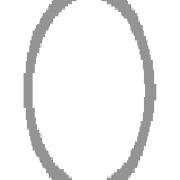
# Autodesk Inventor part: 4130_1x0.065
Saved by Autodesk Inventor 2021 (Build 250183000, 183)
## iProperties
Created: 2020-11-09
Part Number: 4130_1x0.065
Material: Steel, Alloy
Document SubType Name: Modeling
Designer: qv17m
Language: en-US
Size Designation: (Unnamed 1)
Categories: <MemberInstance><Categories><Category DisplayName="Structural Shapes" InternalName="089c4875-fa83-4c05-b084-43b9cc11f5ed" Mnemonic="GRDR"><CategoryParameter DisplayName="Mass per Length Unit" InternalName="0bb95a10-148f-4027-a459-38d7b056702a" Mnemonic="shpmass"/><CategoryParameter DisplayName="Section Area" InternalName="1ff91680-64b0-4202-b9a3-7fd3f94bba3b" Mnemonic="secarea"/><CategoryParameter DisplayName="Radius of Gyration (x)" InternalName="25778675-03e9-40c1-b6a8-4a9ed693320d" Mnemonic="gyrradx"/><CategoryParameter DisplayName="Torsional Rigidity Modulus" InternalName="26c1ec35-5026-4c63-ad0a-751cf684a536" Mnemonic="torrigmod"/><CategoryParameter DisplayName="Distance of the Center of Gravity X-X" InternalName="26c9bdb8-9c79-4b4f-a92e-8e197583c9c4" Mnemonic="grcendistX"/><CategoryParameter DisplayName="Legacy Member ID" InternalName="340afe4f-75d7-48d3-ab7d-943f3c3da468" Mnemonic="LegacyMemberID"/><CategoryParameter DisplayName="Base Length" InternalName="42e34263-8f20-4d0e-ad48-bf1385b87c24" Mnemonic="shplen"/><CategoryParameter DisplayName="Moment of Inertia (y)" InternalName="4b9f58ea-bced-460e-81ea-3d29ca5a49e3" Mnemonic="inermomy"/><CategoryParameter DisplayName="Moment of Inertia (x)" InternalName="4cd780bc-73d7-43ac-917a-579e5cbd684d" Mnemonic="inermomx"/><CategoryParameter DisplayName="Custom Base Point" InternalName="4f1d1b73-316d-484b-a3df-9cbabb16eb77" Mnemonic="shpBasePoint"/><CategoryParameter DisplayName="Shape Height" InternalName="50274e7d-5ac0-4796-92cb-c59e54983c67" Mnemonic="shpheig"/><CategoryParameter DisplayName="Section Module (y)" InternalName="59eaa5e9-d227-48dc-b6c1-6920f96e0f95" Mnemonic="secmody"/><CategoryParameter DisplayName="Section Designation" InternalName="5a64d034-428d-49c8-ba32-7619764de20f" Mnemonic="shpdes"/><CategoryParameter DisplayName="Section Module (x)" InternalName="72cfad18-cf51-4ed4-aaa7-c6b224f8419f" Mnemonic="secmodx"/><CategoryParameter DisplayName="Torsional Section Modulus" InternalName="7c55a8dc-8844-49f9-a867-cc677b30ec9a" Mnemonic="torsecmod"/><CategoryParameter DisplayName="Shape Width" InternalName="7c717d54-a18f-4666-b4d4-573cce22c62c" Mnemonic="shpwdth"/><CategoryParameter DisplayName="Second Shape Thickness" InternalName="9251a8e1-85fd-4e47-af99-afdb762317d9" Mnemonic="shpthick2"/><CategoryParameter DisplayName="FG Authored" InternalName="9c666724-f362-4ea7-ac62-f6a007de5c69" Mnemonic="shpFGAuto"/><CategoryParameter DisplayName="Distance of the Center of Gravity Y-Y" InternalName="bcc4fb17-7af4-436a-8f8c-d0aa3b0248c5" Mnemonic="grcendistY"/><CategoryParameter DisplayName="Radius of Gyration (y)" InternalName="bfa18ebe-1636-4dbe-8d42-b263e0b73184" Mnemonic="gyrrady"/><CategoryParameter DisplayName="Shape Thickness" InternalName="d109cf76-8eb4-42fc-9800-4409734adc67" Mnemonic="shpthick"/><CategoryParameter DisplayName="Coefficient of Shear Displacement" InternalName="de4c90c6-aaa8-468f-a335-6737b311b5d3" Mnemonic="shdispc"/><Category DisplayName="Round Tubes" InternalName="992db413-5889-4444-87eb-da7d0d4daf07" Mnemonic="TBSHP"><CategoryParameter DisplayName="Radius of Gyration (x)" InternalName="3dee80f9-25b5-4b66-b49a-b691523a1a28" Mnemonic="gyrradx"/><CategoryParameter DisplayName="Section Module (x)" InternalName="60bb9a9e-a6fd-4017-9231-e997b611324d" Mnemonic="secmodx"/><CategoryParameter DisplayName="Section Area" InternalName="74b0e21b-5d01-435e-8002-7f0865b0cc07" Mnemonic="secarea"/><CategoryParameter DisplayName="Shape Thickness" InternalName="b5605888-f14d-4c59-a16a-2ee7d0c8b446" Mnemonic="shpthick"/><CategoryParameter DisplayName="Moment of Inertia (x)" InternalName="f00a3c64-1241-4bd0-be8c-851e710b5594" Mnemonic="inermomx"/></Category></Category><Category DisplayName="DataType" InternalName="23b78d0f-2648-40c6-8793-ca6db495c9e8" Mnemonic="DATATYPE"><CategoryParameter DisplayName="DisplayName" InternalName="05415f3d-3907-474b-a020-eb9d644f4cf3" Mnemonic="DISPLAYNAME"/><CategoryParameter DisplayName="Standard" InternalName="0c0a119c-1e12-4c84-803f-101930972f5e" Mnemonic="STANDARD"/><CategoryParameter DisplayName="Description" InternalName="13903e3d-64b1-4950-80da-f627842ea37f" Mnemonic="DESCRIPTION"/><CategoryParameter DisplayName="Designation" InternalName="2675968c-4ce5-49e0-a4f5-552d29089031" Mnemonic="DESIGNATION"/><CategoryParameter DisplayName="Default Row" InternalName="2af9ec52-faaa-4026-b378-f9fa4afca842" Mnemonic="DEFAULTROW"/><CategoryParameter DisplayName="Folder Name" InternalName="3f06958e-8713-4116-9be7-ed6184ecc97b" Mnemonic="FOLDERNAME"/><CategoryParameter DisplayName="Revision Guid" InternalName="45a75005-10b1-4dfc-8d6d-dfe629f0b93c" Mnemonic="REVISIONGUID"/><CategoryParameter DisplayName="FileName" InternalName="8b46a4cc-9585-4fed-90c3-899f57e09a73" Mnemonic="FILENAME"/><CategoryParameter DisplayName="StdsOrg" InternalName="8f5914e1-4693-403f-8ab5-d37768198c9d" Mnemonic="STDSORG"/><CategoryParameter DisplayName="Family Version" InternalName="914462f6-6e19-4b14-ba84-155b9680b1d0" Mnemonic="FAMILYREVISION"/><CategoryParameter DisplayName="Standard Revision" InternalName="91d5a463-65c2-4fde-b823-3b7fea5e8e17" Mnemonic="STANDARDREVISION"/><CategoryParameter DisplayName="Member Revision" InternalName="a65d44b9-392f-4f4f-857b-e4b3d54996fe" Mnemonic="MEMBERREVISION"/><CategoryParameter DisplayName="ClipFormat" InternalName="bc51e27b-3422-4e78-93ef-cec197ddf230" Mnemonic="CLIPFORMAT"/><CategoryParameter DisplayName="Manufacturer" InternalName="cd6c7a72-a28a-4e50-99a9-2c7f4e13e5ad" Mnemonic="MANUFACTURER"/><CategoryParameter DisplayName="InternalName" InternalName="cf1d0246-76d9-4b4a-8305-fa0409afb5c1" Mnemonic="INTERNALNAME"/><CategoryParameter DisplayName="IsMetric" InternalName="e2385c5b-1ea4-4823-96a8-8de651266ec3" Mnemonic="ISMETRIC"/><Category DisplayName="Part" InternalName="c0e0b642-3bcb-4cc8-9e80-f96d35c4afa4" Mnemonic="PART"><CategoryParameter DisplayName="Part Number" InternalName="016b6077-bfbe-49bd-92c9-d8d59c39c941" Mnemonic="PARTNUMBER"/><CategoryParameter DisplayName="Stock Number" InternalName="4dba7c1c-e26c-444e-836c-b08b433409a8" Mnemonic="STOCKNUMBER"/><CategoryParameter DisplayName="Material Key" InternalName="5c9a8adb-dd2b-4535-b97f-0a94a95fe41f" Mnemonic="MATERIALKEY"/><CategoryParameter DisplayName="Material" InternalName="818a152a-d3c3-49ca-80ee-df7d91421b8e" Mnemonic="MATERIAL"/></Category></Category></Categories><FamilyTemplate Id="4130_1x0.065"><FamilyTemplateParameters><FamilyTemplateParameter ObjectType="kModelParameterObject" ValueType="xs:double" Id="12" ObjectReferenceKey="d2"/><FamilyTemplateParameter ObjectType="kPartComponentDefinitionObject" ValueType="xs:string" Id="23" SubObjectId="Material"/><FamilyTemplateParameter ObjectType="kPropertyObject" ValueType="xs:string" Id="26" ObjectReferenceKey="{32853F0F-3444-11d1-9E93-0060B03C1CA6}" SubObjectId="5"/><FamilyTemplateParameter ObjectType="kPropertyObject" ValueType="xs:string" Id="27" ObjectReferenceKey="{32853F0F-3444-11d1-9E93-0060B03C1CA6}" SubObjectId="52"/></FamilyTemplateParameters></FamilyTemplate><CategoryParameterMap><ParamToTemplateMap><ParamToTemplate CategoryParameter="//CategoryParameter[@InternalName='cf1d0246-76d9-4b4a-8305-fa0409afb5c1']" ConstantValue="8416881d-c1a1-4bff-8a73-3abdcd8f8b8b"/><ParamToTemplate CategoryParameter="//CategoryParameter[@InternalName='45a75005-10b1-4dfc-8d6d-dfe629f0b93c']" ConstantValue="aacdff6d-95cb-4088-bf22-46486a784052"/><ParamToTemplate CategoryParameter="//CategoryParameter[@InternalName='3f06958e-8713-4116-9be7-ed6184ecc97b']" ConstantValue="4130_1x0.065"/><ParamToTemplate CategoryParameter="//CategoryParameter[@InternalName='8f5914e1-4693-403f-8ab5-d37768198c9d']" TemplateParameter="17"/><ParamToTemplate CategoryParameter="//CategoryParameter[@InternalName='0c0a119c-1e12-4c84-803f-101930972f5e']" TemplateParameter="18"/><ParamToTemplate CategoryParameter="//CategoryParameter[@InternalName='91d5a463-65c2-4fde-b823-3b7fea5e8e17']" TemplateParameter="19"/><ParamToTemplate CategoryParameter="//CategoryParameter[@InternalName='cd6c7a72-a28a-4e50-99a9-2c7f4e13e5ad']" TemplateParameter="20"/><ParamToTemplate CategoryParameter="//CategoryParameter[@InternalName='13903e3d-64b1-4950-80da-f627842ea37f']" TemplateParameter="22"/><ParamToTemplate CategoryParameter="//CategoryParameter[@InternalName='05415f3d-3907-474b-a020-eb9d644f4cf3']" ConstantValue="4130_1x0.065"/><ParamToTemplate CategoryParameter="//CategoryParameter[@InternalName='914462f6-6e19-4b14-ba84-155b9680b1d0']" ConstantValue="11"/><ParamToTemplate CategoryParameter="//CategoryParameter[@InternalName='bc51e27b-3422-4e78-93ef-cec197ddf230']" ConstantValue="CF_INVENTOR.STDPARTS"/><ParamToTemplate CategoryParameter="//CategoryParameter[@InternalName='e2385c5b-1ea4-4823-96a8-8de651266ec3']" ConstantValue="false"/><ParamToTemplate CategoryParameter="//CategoryParameter[@InternalName='2af9ec52-faaa-4026-b378-f9fa4afca842']" ConstantValue="1"/><ParamToTemplate CategoryParameter="//CategoryParameter[@InternalName='9c666724-f362-4ea7-ac62-f6a007de5c69']" ConstantValue="1"/><ParamToTemplate CategoryParameter="//CategoryParameter[@InternalName='8b46a4cc-9585-4fed-90c3-899f57e09a73']" ConstantValue="Steel, Alloy"/><ParamToTemplate CategoryParameter="//CategoryParameter[@InternalName='a65d44b9-392f-4f4f-857b-e4b3d54996fe']" ConstantValue="5fcc0559-94cb-451d-a04d-a4c026bf219b"/><ParamToTemplate CategoryParameter="//CategoryParameter[@InternalName='a65d44b9-392f-4f4f-857b-e4b3d54996fe']" ConstantValue="5fcc0559-94cb-451d-a04d-a4c026bf219b"/><ParamToTemplate CategoryParameter="//CategoryParameter[@InternalName='2675968c-4ce5-49e0-a4f5-552d29089031']" TemplateParameter="27"/><ParamToTemplate CategoryParameter="//CategoryParameter[@InternalName='818a152a-d3c3-49ca-80ee-df7d91421b8e']" TemplateParameter="23"/><ParamToTemplate CategoryParameter="//CategoryParameter[@InternalName='016b6077-bfbe-49bd-92c9-d8d59c39c941']" TemplateParameter="26"/><ParamToTemplate CategoryParameter="//CategoryParameter[@InternalName='42e34263-8f20-4d0e-ad48-bf1385b87c24']" TemplateParameter="12"/></ParamToTemplateMap></CategoryParameterMap></MemberInstance>
Density: 7.73 g/cm^3
Appearance: Semi-Polished
_CCFamilyDisplayName: 4130_1x0.065
_FrameMemberDoc: Frame Member File
_Version: 25.0.0
_GetPNFromCC: 1
IsCustomPart: 1
G_L: 20.000 in
G_W: 1.000 in
G_H: 1.000 in
+12C06B5C-5AC8-49B0-9636-28DAB5015227+CUTDETAIL1: Notch
+42C8F8DD-CB0E-4885-AC75-E5F940155F2A+CUTDETAIL2: Notch
Author: qv17m
Autodesk Inventor part; units mm, degrees
ref_plane "Start Plane" through (0, 0, 0) normal (1, 0, 0) x (0, 1, 0)
ref_plane "End Plane" through (508, 0, 0) normal (1, 0, 0) x (0, 1, 0)
sketch "Sketch" plane through (0, 0, 0) normal (1, 0, 0) x (0, 1, 0)
  circle A0 centre (0, 0) radius 12.7
  circle A1 centre (0, 0) radius 11.049
  dimension "d0" = 25.4
  dimension "d1" = 1.651
  constraints: 2 centre point, 2 coincident
  measures "d0" diameter of A0
  measures "d1" radial gap between concentric circles of A0 A1
extrude "Body" add sketch "Sketch" along normal up to surface (508 mm away) from surface at 0
sketch "Sketch2" plane through (0, 0, 0) normal (1, 0, 0) x (0, 1, 0)
  line L0 (0, 0) -> (10, 0)
ref_plane "Work Plane3" through (0, 0, 0) normal (0, 0, -1) x (0, 1, 0)
sketch "Sketch3" plane through (0, 0, 0) normal (0, 0, -1) x (0, 1, 0)
  line L0 (-2, 0) -> (12, 0)
  line L1 (-2, 508) -> (12, 508)
  dimension "d9" = 508
  measures "d9" distance between parallel lines of L0 L1
ref_plane "Work Plane4" through (508, -502.927704, -71.608135) normal (0, 0.9900152, 0.1409609) x (0.421359, -0.1278366, 0.8978388)
ref_plane "Work Plane5" through (508, 12.573193, 1.790203) normal (0, 0.9900152, 0.1409609) x (0.421359, -0.1278366, 0.8978388)
ref_plane "Work Plane6" through (508, -245.177255, -34.908966) normal (0, 0.9900152, 0.1409609) x (0.9068939, 0.0593951, -0.4171518)
sketch "Sketch4" plane through (508, -245.177255, -34.908966) normal (0, 0.9900152, 0.1409609) x (0.9068939, 0.0593951, -0.4171518)
  circle A0 centre (0, 0) radius 12.7
  circle A1 centre (0, 0) radius 11.049
  constraints: 2 centre point
extrude "Extrusion3" add sketch "Sketch4" along normal up to surface (520.7 mm away) from surface at -260.35 separate body contours A0 | A1
combine bodies "Combine1" operation type subtract main body 1 bodies to subtract 2
ref_plane "Work Plane7" through (0, 12.573193, 1.790203) normal (0, -0.9900152, -0.1409609) x (-0.7758461, 0.0889354, -0.6246225)
ref_plane "Work Plane8" through (0, -502.927704, -71.608135) normal (0, -0.9900152, -0.1409609) x (-0.7758461, 0.0889354, -0.6246225)
ref_plane "Work Plane9" through (0, -245.177255, -34.908966) normal (0, -0.9900152, -0.1409609) x (0.6309222, 0.109364, -0.7680994)
sketch "Sketch5" plane through (0, -245.177255, -34.908966) normal (0, -0.9900152, -0.1409609) x (0.6309222, 0.109364, -0.7680994)
  circle A0 centre (0, 0) radius 12.7
  circle A1 centre (0, 0) radius 11.049
  constraints: 2 centre point
extrude "Extrusion4" add sketch "Sketch5" along normal up to surface (520.7 mm away) from surface at -260.35 separate body contours A0 | A1
combine bodies "Combine2" operation type subtract main body 1 bodies to subtract 3
equation "\"G_OFFSET_START\" = 0"
equation "\"G_OFFSET_END\" = 0"
equation "\"d5\" = d2 + G_OFFSET_END"
equation "\"G_L\" = d9"
equation "\"d2\" = 508"
body "Solid1"
